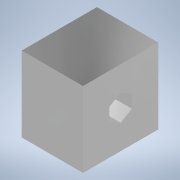
# Autodesk Inventor part: Cubo
Saved by Autodesk Inventor 2022.1 (Build 261234000, 234)
## iProperties
Part Number: Cubo
Material: Aluminio 6061
Document SubType Name: Modelado
Designer: seb_0
Appearance: Aluminio - Plano
Density: 2.7 g/cm^3
Author: seb_0
Autodesk Inventor part; units mm, degrees
ref_plane "Plano YZ" through (0, 0, 0) normal (1, 0, 0) x (0, 1, 0)
ref_plane "Plano XZ" through (0, 0, 0) normal (0, 1, 0) x (-1, 0, 0)
ref_plane "Plano XY" through (0, 0, 0) normal (0, 0, 1) x (1, 0, 0)
sketch "Boceto1" plane through (0, 0, 0) normal (1, 0, 0) x (0, 1, 0)
  circle A0 centre (0, 0) radius 1.7
  circle A1 centre (0, 0) radius 9.2
  line L0 (9.2, 9.2) -> (-9.2, 9.2)
  line L1 (-9.2, 9.2) -> (-9.2, -9.2)
  line L2 (-9.2, -9.2) -> (9.2, -9.2)
  line L3 (9.2, -9.2) -> (9.2, 9.2)
  dimension "d0" = 3.4
  dimension "d2" = 7.5
  constraints: 8 end point, 4 tangent, 2 centre point, 2 parallel, 1 coincident, 1 horizontal, 1 perpendicular
  measures "d0" diameter of A0
  measures "d2" radial gap between concentric circles of A0 A1
extrude "Extrusión1" add sketch "Boceto1" along normal blind 15
sketch "Boceto2" plane through (15, 0, 0) normal (1, 0, 0) x (0, 0, -1)
  line L0 (2.7496, -1.5875) -> (0, -3.175)
  line L1 (0, -3.175) -> (-2.7496, -1.5875)
  line L2 (-2.7496, -1.5875) -> (-2.7496, 1.5875)
  line L3 (-2.7496, 1.5875) -> (0, 3.175)
  line L4 (0, 3.175) -> (2.7496, 1.5875)
  line L5 (2.7496, 1.5875) -> (2.7496, -1.5875)
  point P0 (0, 0)
  point P1 (0, 0)
  dimension "d5" = 3.175
  constraints: 12 end point, 1 coincident, 1 vertical, 13 other
  measures "d5" distance of L4.end L0.start
extrude "Extrusión2" cut sketch "Boceto2" against normal blind 10
